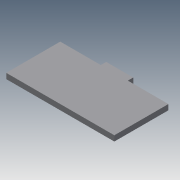
# Autodesk Inventor part: MoistureBeatrobo2l
Saved by Autodesk Inventor 2014 (Build 180170000, 170)
## iProperties
Created: 2014-06-14
Part Number: MoistureBeatrobo2l
Material: 一般
Document SubType Name: Modeling
Designer: Hideyuki Takei
Density: 1 g/cm^3
Appearance: 既定
Author: Hideyuki Takei
Autodesk Inventor part; units mm, degrees
ref_plane "YZ Plane" through (0, 0, 0) normal (1, 0, 0) x (0, 1, 0)
ref_plane "XZ Plane" through (0, 0, 0) normal (0, 1, 0) x (-1, 0, 0)
ref_plane "XY Plane" through (0, 0, 0) normal (0, 0, 1) x (1, 0, 0)
sketch "スケッチ1" plane through (0, 0, 0) normal (0, 0, 1) x (1, 0, 0)
  line L0 (0, 0) -> (40, 0)
  line L1 (40, 0) -> (40, 20)
  line L2 (40, 20) -> (0, 20)
  line L3 (0, 20) -> (0, 0)
  line L4 (15, 20) -> (25, 20)
  line L5 (25, 20) -> (25, 22)
  line L6 (25, 22) -> (15, 22)
  line L7 (15, 22) -> (15, 20)
  dimension "d0" = 20
  dimension "d1" = 40
  dimension "d2" = 10
  dimension "d3" = 2
  dimension "d4" = 20
  dimension "d5" = 15
  constraints: 16 end point, 4 parallel, 2 horizontal, 2 perpendicular
  measures "d0" distance of L2.end L0.start
  measures "d1" distance of L1.end L2.end
  measures "d2" distance of L5.end L6.end
  measures "d3" distance of L6.end L4.start
  measures "d4" distance between parallel lines of L0 L4
  measures "d5" distance between parallel lines of L3 L7
extrude "押し出し1" add sketch "スケッチ1" along normal blind 2
